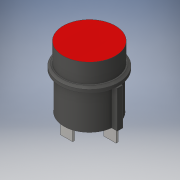
# Autodesk Inventor part: SwitchPushButton
Saved by Autodesk Inventor 2016 (Build 200138000, 138)
## iProperties
Created: 2015-10-16
Part Number: SwitchPushButton
Material: Generic
Document SubType Name: Modeling
Designer: lachesis
Density: 1 g/cm^3
Appearance: Default
Author: lachesis
Autodesk Inventor part; units mm, degrees
ref_plane "YZ Plane" through (0, 0, 0) normal (1, 0, 0) x (0, 1, 0)
ref_plane "XZ Plane" through (0, 0, 0) normal (0, 1, 0) x (-1, 0, 0)
ref_plane "XY Plane" through (0, 0, 0) normal (0, 0, 1) x (1, 0, 0)
sketch "Sketch1" plane through (0, 0, 0) normal (0, 1, 0) x (-1, 0, 0)
  circle A0 centre (0, 0) radius 9.9
  line L0 (-9.8387, 1.1) -> (-12.0387, 1.1)
  line L1 (-12.0387, 1.1) -> (-12.0387, -1.1)
  line L2 (-12.0387, -1.1) -> (-9.8387, -1.1)
  point P0 (-12.0387, 0)
  dimension "d0" = 19.8
  dimension "d1" = 2.2
  dimension "d2" = 2.2
  constraints: 6 end point, 2 perpendicular, 2 point on circle, 1 centre point, 1 coincident, 1 horizontal, 1 horizontal alignment, 1 midpoint, 1 parallel
  measures "d0" diameter of A0
  measures "d1" distance of L0.end L1.end
  measures "d2" distance of L1.end L2.end
extrude "Extrusion1" add sketch "Sketch1" along normal blind 14.5
sketch "Sketch2" plane through (0, 14.5, 0) normal (0, 1, 0) x (1, 0, 0)
  circle A0 centre (0, 0) radius 11.5
  dimension "d5" = 23
  constraints: 1 centre point, 1 coincident
  measures "d5" diameter of A0
extrude "Extrusion2" add sketch "Sketch2" along normal blind 2
chamfer "Chamfer1" distance 0.8 angle 45 1 edges at (-11.5, 16.5, 0)
sketch "Sketch3" plane through (0, 16.5, 0) normal (0, 1, 0) x (1, 0, 0)
  circle A0 centre (0, 0) radius 10.2
  dimension "d11" = 20.4
  constraints: 1 centre point, 1 coincident
  measures "d11" diameter of A0
extrude "Extrusion3" add sketch "Sketch3" along normal blind 7.5
sketch "Sketch4" plane through (0, 0, 0) normal (0, -1, 0) x (1, 0, 0)
  line L0 (-6.875, -4.4) -> (-2.125, -4.4)
  line L1 (-2.125, -4.4) -> (-2.125, -3.6)
  line L2 (-2.125, -3.6) -> (-6.875, -3.6)
  line L3 (-6.875, -3.6) -> (-6.875, -4.4)
  line L4 (2.125, -4.4) -> (6.875, -4.4)
  line L5 (6.875, -4.4) -> (6.875, -3.6)
  line L6 (6.875, -3.6) -> (2.125, -3.6)
  line L7 (2.125, -3.6) -> (2.125, -4.4)
  line L8 (-6.875, 3.6) -> (-2.125, 3.6)
  line L9 (-2.125, 3.6) -> (-2.125, 4.4)
  line L10 (-2.125, 4.4) -> (-6.875, 4.4)
  line L11 (-6.875, 4.4) -> (-6.875, 3.6)
  line L12 (-4.5, -3.6) -> (-4.5, 3.6)
  line L13 (2.125, -4) -> (-2.125, -4)
  point P0 (0, 0)
  point P1 (-4.5, -4.4)
  point P2 (4.5, -4.4)
  point P3 (-2.125, 4)
  point P4 (-4.5, 0)
  point P5 (0, -4)
  dimension "d14" = 0.8
  dimension "d15" = 4.75
  dimension "d16" = 9
  dimension "d17" = 8
  constraints: 28 end point, 9 midpoint, 6 parallel, 4 perpendicular, 4 point on line, 3 horizontal, 2 collinear, 1 horizontal alignment, 1 vertical alignment
  measures "d14" distance of L0.end L1.end
  measures "d15" distance of L0.start L0.end
  measures "d16" distance of point (4.5, -4.4) point (-4.5, -4.4)
  measures "d17" distance of point (-2.125, 4) L13.end
extrude "Extrusion4" add sketch "Sketch4" along normal blind 9
equation "\"d2\" = d1"
body "Solid1"
